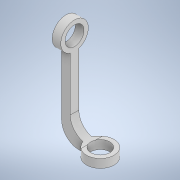
# Autodesk Inventor part: Gora-srodek-ramie
Saved by Autodesk Inventor 2022 (Build 260153000, 153)
## iProperties
Created: 2022-03-27
Part Number: Gora-srodek-ramie
Material: Ogólny
Document SubType Name: Modeling
Designer: jolow
Density: 1 g/cm^3
Appearance: Domyślna
Author: jolow
Autodesk Inventor part; units mm, degrees
ref_plane "YZ Plane" through (0, 0, 0) normal (1, 0, 0) x (0, 1, 0)
ref_plane "XZ Plane" through (0, 0, 0) normal (0, 1, 0) x (-1, 0, 0)
ref_plane "XY Plane" through (0, 0, 0) normal (0, 0, 1) x (1, 0, 0)
sketch "Szkic2" plane through (0, 0, 0) normal (0, 1, 0) x (-1, 0, 0)
  circle A0 centre (0, 0) radius 11
  circle A1 centre (0, 0) radius 16
  dimension "d0" = 22
  dimension "d1" = 5
  constraints: 2 centre point, 2 coincident
  measures "d0" diameter of A0
  measures "d1" radial gap between concentric circles of A0 A1
extrude "Wyciągnięcie proste1" add sketch "Szkic2" along normal blind 10
sketch "Szkic4" plane through (0, 0, 0) normal (0, 0, 1) x (1, 0, 0)
  line L0 (0, 0) -> (-30, 0)
  line L1 (-30, 0) -> (-30, 10)
  line L2 (-30, 10) -> (0, 10)
  line L3 (0, 10) -> (0, 0)
  line L4 (-30, 0) -> (-40, 0)
  line L5 (-40, 0) -> (-40, 107.5)
  line L6 (-40, 107.5) -> (-30, 107.5)
  line L7 (-30, 107.5) -> (-30, 0)
  dimension "d7" = 107.5
  dimension "d8" = 30
  dimension "d9" = 10
  dimension "d10" = 10
  constraints: 16 end point, 4 parallel, 2 horizontal, 2 perpendicular
  measures "d7" distance of L4.end L5.end
  measures "d8" distance of L1.end L2.end
  measures "d9" distance of L5.end L6.end
  measures "d10" distance of L2.end L0.start
extrude "Wyciągnięcie proste2" add sketch "Szkic4" along normal mid plane 10
fillet "Zaokrąglenie1" radius 20 2 edges at (-40, 0, 0) (-30, 10, 0)
sketch "Szkic7" plane through (-30, 107.5, 5) normal (1, 0, 0) x (0, 0, -1)
  line L0 (10, 0) -> (0, 0) projected
  circle A0 centre (5, 0) radius 11
  circle A1 centre (5, 0) radius 16
  point P0 (5, -107.5)
  dimension "d14" = 22
  dimension "d15" = 32
  constraints: 2 centre point, 1 coincident, 1 midpoint
  measures "d14" diameter of A0
  measures "d15" diameter of A1
extrude "Wyciągnięcie proste3" add sketch "Szkic7" against normal blind 10
sketch "Szkic8" plane through (0, 10, 0) normal (0, 1, 0) x (1, 0, 0)
  circle A0 centre (0, 0) radius 11
  constraints: 1 centre point, 1 coincident
extrude "Wyciągnięcie proste4" cut sketch "Szkic8" against normal blind 10
sketch "Szkic9" plane through (0, 10, 0) normal (0, -1, 0) x (1, 0, 0)
  circle A0 centre (0, 0) radius 11
  constraints: 1 centre point, 1 coincident
extrude "Wyciągnięcie proste5" cut sketch "Szkic9" against normal blind 10
sketch "Szkic11" plane through (-30, 30, 5) normal (1, 0, 0) x (0, 0, -1)
  line L0 (10, 77.5) -> (0, 77.5) projected
  circle A0 centre (5, 77.5) radius 11
  point P0 (5, -30)
  constraints: 1 centre point, 1 midpoint
extrude "Wyciągnięcie proste6" cut sketch "Szkic11" against normal blind 10
